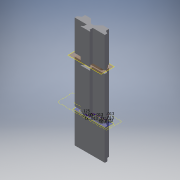
# Autodesk Inventor part: Holder_Slide
Saved by Autodesk Inventor 2019 (Build 230136000, 136)
## iProperties
Created: 2021-01-21
Part Number: Holder_Slide
Material: Generic
Document SubType Name: Modeling
Designer: zhanb
Density: 1 g/cm^3
Appearance: Default
Author: zhanb
Autodesk Inventor part; units mm, degrees
ref_plane "YZ Plane" through (0, 0, 0) normal (1, 0, 0) x (0, 1, 0)
ref_plane "XZ Plane" through (0, 0, 0) normal (0, 1, 0) x (-1, 0, 0)
ref_plane "XY Plane" through (0, 0, 0) normal (0, 0, 1) x (1, 0, 0)
sketch "Sketch1" plane through (0, 0, 0) normal (0, 1, 0) x (-1, 0, 0)
  line L0 (12.7, -15.875) -> (12.7, -12.7) construction
  line L1 (12.7, -12.7) -> (15.875, -10.8669) construction
  line L2 (15.875, -10.8669) -> (15.875, -7.9375) construction
  line L3 (15.875, -7.9375) -> (6.35, -7.9375) construction
  line L4 (6.35, -7.9375) -> (6.35, -3.175) construction
  line L5 (6.35, -3.175) -> (3.175, -3.175) construction
  line L6 (3.175, -3.175) -> (3.175, -6.35) construction
  line L7 (3.175, -6.35) -> (4.7625, -7.2665) construction
  line L8 (4.7625, -7.2665) -> (4.7625, -7.9375) construction
  line L9 (4.7625, -7.9375) -> (-4.7625, -7.9375) construction
  line L10 (-4.7625, -7.9375) -> (-4.7625, -7.2665) construction
  line L11 (-4.7625, -7.2665) -> (-3.175, -6.35) construction
  line L12 (-3.175, -6.35) -> (-3.175, -3.175) construction
  line L13 (-3.175, -3.175) -> (-6.35, -3.175) construction
  line L14 (-6.35, -3.175) -> (-6.35, -7.9375) construction
  line L15 (-6.35, -7.9375) -> (-15.875, -7.9375) construction
  line L16 (-15.875, -7.9375) -> (-15.875, -10.8669) construction
  line L17 (-15.875, -10.8669) -> (-12.7, -12.7) construction
  line L18 (-12.7, -12.7) -> (-12.7, -15.875) construction
  line L19 (-25.4, -15.875) -> (-12.7, -15.875) construction
  line L20 (-25.4, 0) -> (-25.4, -15.875) construction
  line L21 (25.4, 0) -> (-25.4, 0) construction
  line L22 (25.4, 0) -> (25.4, -15.875) construction
  line L23 (12.7, -15.875) -> (25.4, -15.875) construction
  line L24 (-12.3825, -15.875) -> (-12.3825, -12.5167)
  line L25 (-12.3825, -12.5167) -> (-15.5575, -10.6836)
  line L26 (-15.5575, -10.6836) -> (-15.5575, -8.255)
  line L27 (-15.5575, -8.255) -> (-6.0325, -8.255)
  line L28 (-6.0325, -8.255) -> (-6.0325, -3.4925) construction
  line L29 (-12.3825, -15.875) -> (0, -15.875)
  line L30 (0, -15.875) -> (0, -8.255)
  line L31 (-6.0325, -8.255) -> (0, -8.255)
  line L32 (0, -8.255) -> (0, -3.4925)
  line L33 (-3.175, -8.255) -> (-3.175, -5.08)
  line L34 (-3.175, -5.08) -> (-4.7625, -4.1635)
  line L35 (-4.7625, -4.1635) -> (-4.7625, -3.4925)
  line L36 (-6.0325, -3.4925) -> (-4.7625, -3.4925) construction
  line L37 (-4.7625, -3.4925) -> (0, -3.4925)
  point P0 (0, -7.9375)
  dimension "d1" = 0.3175
  dimension "d2" = 0.3175
  dimension "d3" = 0.3175
  dimension "d4" = 0.3175
  dimension "d5" = 0.3175
  dimension "d12" = 3.175
  dimension "d13" = 0.3175
  dimension "d14" = 30
  constraints: 28 end point, 6 vertical, 4 horizontal, 4 point on line, 3 collinear, 2 parallel, 1 midpoint
  measures "d1" distance between parallel lines of L18 L24
  measures "d2" distance between parallel lines of L17 L25
  measures "d3" distance between parallel lines of L16 L26
  measures "d4" distance between parallel lines of L27 L15
  measures "d5" distance between parallel lines of L14 L28
  measures "d12" distance of L33.start L33.end
  measures "d13" distance between parallel lines of L13 L36
  measures "d14" angle of L37 L34
extrude "Extrusion1" add sketch "Sketch1" along normal blind 76.2
extrude "Extrusion2" add sketch "Sketch1" against normal blind 38.1 contours L24 L25 L26 L27 L31 L30 L29
mirror "Mirror1" about plane through (0, 0, -8.255) normal (-1, 0, 0) of "Extrusion1", "Extrusion2"
sketch "Sketch2" plane through (0, -38.1, 0) normal (0, -1, 0) x (1, 0, 0)
  line L0 (12.3825, -15.875) -> (-12.3825, -15.875) construction
  line L1 (12.3825, -15.875) -> (12.3825, -12.5167) construction
  line L2 (12.3825, -12.5167) -> (15.5575, -10.6836) construction
  line L3 (15.5575, -10.6836) -> (15.5575, -8.255) construction
  line L4 (15.5575, -8.255) -> (-15.5575, -8.255) construction
  line L5 (-15.5575, -10.6836) -> (-15.5575, -8.255) construction
  line L6 (-12.3825, -12.5167) -> (-15.5575, -10.6836) construction
  line L7 (-12.3825, -15.875) -> (-12.3825, -12.5167) construction
  circle A0 centre (0, -16.6845) radius 5.08 construction
  line L8 (12.3825, -15.875) -> (-12.3825, -15.875) construction
  line L9 (6.2865, -15.875) -> (1.5875, -11.176)
  line L10 (1.5875, -11.176) -> (-1.5875, -11.176)
  line L11 (-1.5875, -11.176) -> (-6.2865, -15.875)
  line L12 (0, -11.176) -> (0, -15.875) construction
  line L13 (6.2865, -15.875) -> (-6.2865, -15.875)
  point P0 (0, 0)
  dimension "d15" = 10.16
  dimension "d16" = 4.699
  dimension "d17" = 45
  dimension "d18" = 3.175
  constraints: 10 end point, 2 midpoint, 2 point on line, 1 centre point, 1 collinear, 1 parallel, 1 vertical, 1 vertical alignment, 1 other
  measures "d15" diameter of A0
  measures "d16" distance between parallel lines of L0 L10
  measures "d17" angle of L0 L9
  measures "d18" distance of L9.end L10.end
extrude "Extrusion3" cut sketch "Sketch2" against normal through all
ref_plane "Work Plane1" through (0, -6.35, 0) normal (0, -1, 0) x (1, 0, 0)
sketch "Sketch3" plane through (0, -6.35, 0) normal (0, -1, 0) x (1, 0, 0)
  line L0 (-6.2865, -15.875) -> (-1.5875, -11.176) construction
  line L1 (-1.5875, -11.176) -> (1.5875, -11.176) projected
  line L2 (1.5875, -11.176) -> (6.2865, -15.875) construction
  line L3 (12.3825, -15.875) -> (6.2865, -15.875) construction
  line L4 (12.3825, -15.875) -> (12.3825, -12.5167) projected
  line L5 (12.3825, -12.5167) -> (15.5575, -10.6836) projected
  line L6 (15.5575, -10.6836) -> (15.5575, -8.255) projected
  line L7 (15.5575, -8.255) -> (-15.5575, -8.255) construction
  line L8 (-15.5575, -10.6836) -> (-15.5575, -8.255) projected
  line L9 (-12.3825, -12.5167) -> (-15.5575, -10.6836) projected
  line L10 (-12.3825, -15.875) -> (-12.3825, -12.5167) projected
  line L11 (-6.2865, -15.875) -> (-12.3825, -15.875) projected
  line L12 (12.3825, -15.875) -> (6.2865, -15.875) construction
  line L13 (11.3665, -15.875) -> (11.3665, -11.9301)
  line L14 (11.3665, -11.9301) -> (14.5415, -10.097) construction
  line L15 (14.5415, -10.097) -> (14.5415, -9.271) construction
  line L16 (14.5415, -9.271) -> (10.0965, -9.271) construction
  line L17 (0, -9.271) -> (0, -11.176) construction
  line L18 (1.5875, -11.176) -> (-1.5875, -11.176) projected
  line L19 (12.3825, -15.875) -> (11.3665, -15.875)
  line L20 (0, -9.271) -> (0, -8.255)
  line L21 (-3.175, -8.255) -> (3.175, -8.255) construction
  line L22 (15.5575, -8.255) -> (0, -8.255)
  line L23 (11.3665, -11.9301) -> (11.3665, -10.541)
  line L24 (11.3665, -10.541) -> (10.0965, -9.271)
  line L25 (10.0965, -9.271) -> (0, -9.271)
  point P0 (0, 0)
  dimension "d22" = 1.016
  dimension "d23" = 1.016
  dimension "d24" = 1.016
  dimension "d25" = 1.016
  dimension "d26" = 45
  dimension "d27" = 1.27
  constraints: 22 end point, 5 perpendicular, 3 midpoint, 2 collinear, 1 parallel, 1 point on line
  measures "d22" distance between parallel lines of L13 L4
  measures "d23" distance between parallel lines of L5 L14
  measures "d24" distance between parallel lines of L6 L15
  measures "d25" distance between parallel lines of L7 L16
  measures "d26" angle of L16 L24
  measures "d27" distance from line of L16 L23.end
extrude "Extrusion4" cut sketch "Sketch3" against normal blind 3.175
ref_plane "Work Plane2" through (0, 44.45, 0) normal (0, 1, 0) x (1, 0, 0)
sketch "Sketch4" plane through (0, 44.45, 0) normal (0, 1, 0) x (1, 0, 0)
  line L0 (-1.5875, 11.176) -> (-6.2865, 15.875) construction
  line L1 (-6.2865, 15.875) -> (-12.3825, 15.875) construction
  line L2 (-12.3825, 12.5167) -> (-12.3825, 15.875) construction
  line L3 (-15.5575, 10.6836) -> (-12.3825, 12.5167) construction
  line L4 (-15.5575, 8.255) -> (-15.5575, 10.6836) construction
  line L5 (-3.175, 8.255) -> (-15.5575, 8.255) construction
  line L6 (-3.175, 5.08) -> (-3.175, 8.255) construction
  line L7 (-4.7625, 4.1635) -> (-3.175, 5.08) construction
  line L8 (-4.7625, 3.4925) -> (-4.7625, 4.1635) construction
  line L9 (4.7625, 3.4925) -> (-4.7625, 3.4925) construction
  line L10 (4.7625, 3.4925) -> (4.7625, 4.1635) projected
  line L11 (4.7625, 4.1635) -> (3.175, 5.08) projected
  line L12 (3.175, 5.08) -> (3.175, 8.255) projected
  line L13 (3.175, 8.255) -> (15.5575, 8.255) projected
  line L14 (15.5575, 8.255) -> (15.5575, 10.6836) projected
  line L15 (15.5575, 10.6836) -> (12.3825, 12.5167) projected
  line L16 (12.3825, 12.5167) -> (12.3825, 15.875) projected
  line L17 (12.3825, 15.875) -> (6.2865, 15.875) construction
  line L18 (6.2865, 15.875) -> (1.5875, 11.176) construction
  line L19 (1.5875, 11.176) -> (-1.5875, 11.176) construction
  line L20 (12.3825, 15.875) -> (6.2865, 15.875) construction
  line L21 (11.3665, 15.875) -> (11.3665, 10.541)
  line L22 (11.3665, 10.541) -> (10.0965, 9.271)
  line L23 (10.0965, 9.271) -> (0, 9.271)
  line L24 (0, 9.271) -> (0, 3.4925)
  line L25 (4.7625, 3.4925) -> (-4.7625, 3.4925) construction
  line L26 (12.3825, 15.875) -> (11.3665, 15.875)
  line L27 (4.7625, 3.4925) -> (0, 3.4925)
  point P0 (0, 0)
  dimension "d37" = 1.016
  dimension "d38" = 45
  dimension "d39" = 1.016
  dimension "d40" = 1.27
  constraints: 12 end point, 3 perpendicular, 2 collinear, 1 midpoint, 1 point on line
  measures "d37" distance between parallel lines of L16 L21
  measures "d38" angle of L23 L22
  measures "d39" distance between parallel lines of L13 L23
  measures "d40" distance from line of L23 L21.end
extrude "Extrusion5" cut sketch "Sketch4" against normal blind 3.175
mirror "Mirror2" about plane through (0, 0, 0) normal (1, 0, 0) of "Extrusion4", "Extrusion5"
equation "\"d2\" = d1"
equation "\"d3\" = d1"
equation "\"d4\" = d1"
equation "\"d5\" = d1"
equation "\"d13\" = d1"
equation "\"d23\" = d22"
equation "\"d24\" = d22"
equation "\"d25\" = d22"
equation "\"d37\" = d22"
equation "\"d39\" = d22"
body "Solid1"
